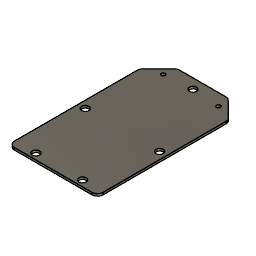
base_piso_3_carga (Autodesk Fusion 360 design; units mm, degrees)
Autodesk Fusion 360 part; units mm, degrees
imported_body "Operación base derivada4" makes body 1
imported_body "Operación base derivada5" makes body 2
imported_body "Operación base derivada6" makes body 3
imported_body "Operación base derivada7" makes body 4
imported_body "Operación base derivada8" makes body 5
sketch "Boceto1" plane through (0, 0, 0) normal (0, 0, 1) x (1, 0, 0)
  line L0 (-80.1041, -35.0015) -> (-80.1041, -116.4458)
  line L1 (-0.0741, 152.5) -> (-0.0741, -130) construction
  line L2 (-80, 72.5) -> (80.1608, 72.5) construction
  arc A0 (-78.7959, 73.6379) -> (-79.0142, 70.8179) centre (-77.4951, 72.1188) ccw
  line L3 (-120, 0) -> (120, 0) construction
  arc A1 (78.866, 70.8179) -> (78.6478, 73.6379) centre (77.3469, 72.1188) ccw
  line L4 (-77.1752, 112.3118) -> (-48.2759, 141.2111)
  line L5 (-83.6742, 105.8127) -> (-54.7157, 105.8127) construction
  line L6 (-80.1041, 32.4265) -> (-80.1041, -35.0015)
  arc A2 (-42.619, 143.5542) -> (-48.2759, 141.2111) centre (-42.619, 135.5542) ccw
  circle A3 centre (-30.0741, 135.5542) radius 3.5 construction
  circle A4 centre (-67.1041, 23.5542) radius 6.5 construction
  circle A5 centre (-67.1041, -115.4458) radius 6.5 construction
  circle A6 centre (29.9259, 135.5542) radius 3.5 construction
  circle A7 centre (66.9559, 23.5542) radius 6.5 construction
  line L7 (-80.1041, 32.4265) -> (-80.1041, 105.2407)
  arc A8 (-77.1752, 112.3118) -> (-80.1041, 105.2407) centre (-70.1041, 105.2407) ccw
  arc A9 (48.1277, 141.2111) -> (42.4708, 143.5542) centre (42.4708, 135.5542) ccw
  line L8 (-42.619, 143.5542) -> (42.4708, 143.5542)
  arc A10 (79.9559, 105.2407) -> (77.027, 112.3118) centre (69.9559, 105.2407) ccw
  line L9 (77.027, 112.3118) -> (48.1277, 141.2111)
  line L10 (79.9559, 32.4265) -> (79.9559, 105.2407)
  line L11 (79.9559, 32.4265) -> (79.9559, -35.0015)
  line L12 (79.9559, -35.0015) -> (79.9559, -116.4458)
  line L13 (-70.1041, -126.4458) -> (69.9559, -126.4458)
  arc A11 (69.9559, -126.4458) -> (79.9559, -116.4458) centre (69.9559, -116.4458) ccw
  arc A12 (-80.1041, -116.4458) -> (-70.1041, -126.4458) centre (-70.1041, -116.4458) ccw
  circle A13 centre (66.9559, -115.4458) radius 6.5 construction
  circle A14 centre (-49.8718, 121.9877) radius 3.5
  circle A15 centre (29.9259, 135.5542) radius 3.5 construction
  circle A16 centre (49.7236, 121.9877) radius 3.5
  circle A17 centre (-67.1041, -1.4458) radius 6.5
  circle A18 centre (66.9559, -1.4458) radius 6.5
  circle A19 centre (-42.1041, -115.4458) radius 6.5
  circle A20 centre (41.9559, -115.4458) radius 6.5
  circle A21 centre (-0.0741, 125.5542) radius 6.5
  point P0 (-45.8598, 143.6271)
  point P1 (47.4167, 143.5198)
  point P2 (-82.9449, -126.3729)
  dimension "d14" = 2
  dimension "d54" = 45
  dimension "d109" = 8
  dimension "d116" = 7
  dimension "d118" = 30
  dimension "d119" = 13
  dimension "d120" = 13
  dimension "d122" = 13
  dimension "d132" = 13
  dimension "d137" = 10
  dimension "d140" = 80.03
  dimension "d141" = 10
  dimension "d142" = 10
  dimension "d143" = 8
  dimension "d144" = 11
  dimension "d145" = 150
  dimension "d146" = 270
  dimension "d147" = 7
  dimension "d149" = 24
  dimension "d150" = 13
  dimension "d152" = 25
  dimension "d153" = 13
  dimension "d154" = 13
  dimension "d156" = 25
  dimension "d157" = 13
  dimension "d158" = 18
  constraint vertical L0
  constraint symmetric L1 A0.start A1.end
  constraint symmetric L1 A0.end A1.start
  constraint symmetric L1 A0 A1
  constraint horizontal L5
  constraint parallel L0 L6
  constraint coincident L5.start L4
  constraint coincident P0 L4
  constraint tangent L4 A2
  constraint symmetric L1 A3 A6
  constraint symmetric L1 A4 A7
  constraint vertical L7
  constraint tangent L4 A8
  constraint tangent L7 A8
  constraint symmetric L1 A2.start A9.end
  constraint symmetric L1 L4.end A9.start
  constraint symmetric L1 A2 A9
  constraint tangent A9 L8
  constraint symmetric L0.start L1 L11.end
  constraint symmetric L1 L6.start L10.start
  constraint symmetric L1 L4.start A10.end
  constraint symmetric L1 L7.end A10.start
  constraint symmetric L1 A8 A10
  constraint tangent L12 A11
  constraint tangent L13 A11
  constraint tangent L0 A12
  constraint tangent L13 A12
  constraint symmetric L1 A5 A13
  constraint symmetric L1 A3 A15
  constraint symmetric L1 A14 A16
  constraint symmetric L1 A17 A18
  constraint symmetric L1 A19 A20
  constraint coincident L1 A21.centre
  measures "d14" radius of A0
  measures "d54" angle of L4 L5
  measures "d109" radius of A2
  measures "d116" diameter of A3
  measures "d118" distance of L1 A3.centre
  measures "d119" diameter of A4
  measures "d120" distance of L6 A4.centre
  measures "d122" diameter of A5
  measures "d132" distance of L0 A5.centre
  measures "d137" radius of A8
  measures "d140" distance of L0 L1
  measures "d141" radius of A11
  measures "d142" radius of A12
  measures "d143" distance of A3.centre L8
  measures "d144" distance of A5.centre L13
  measures "d145" distance of A4.centre L13
  measures "d146" vertical distance of A2.start L13.start
  measures "d147" diameter of A14
  measures "d149" distance of A3.centre A14.centre
  measures "d150" diameter of A17
  measures "d152" vertical distance of A4.centre A17.centre
  measures "d153" distance of L6 A17.centre
  measures "d154" diameter of A19
  measures "d156" distance of A5.centre A19.centre
  measures "d157" diameter of A21
  measures "d158" distance of L8 A21.centre
extrude "Extruir7" add sketch "Boceto1" along normal blind 4 separate body makes body 6
hidden bodies 1 2 3 4 5
named bodies: "Cuerpo1 (Contexto3)", "Cuerpo1 (1) (Contexto3)", "Cuerpo1 (2) (Contexto3)", "Cuerpo1 (3) (Contexto3)", "Cuerpo1 (4) (Contexto3)"
